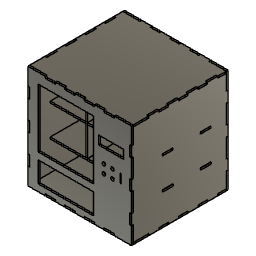
SAVEnding_CAD (Autodesk Fusion 360 design; units mm, degrees)
Autodesk Fusion 360 part; units mm, degrees
note: some values were not read from the file. Set by a fixed rule: which sketch regions a step uses.
(part 1 of 2)
sketch "Sketch3" plane through (0, 0, 0) normal (0, 1, 0) x (1, 0, 0)
  line L0 (0, 0) -> (300, 0)
  line L1 (300, 0) -> (300, -300)
  line L2 (300, -300) -> (0, -300)
  line L3 (0, -300) -> (0, 0)
  dimension "d9" = 300
  dimension "d10" = 300
  constraint horizontal L0
  constraint vertical L1
  constraint horizontal L2
  constraint vertical L3
  constraint coincident L0.start L3.end
  measures "d9" distance of L0.start L0.end
  measures "d10" distance of L0.start L2.end
extrude "Extrude2" add sketch "Sketch3" along normal blind 5 makes body 1
sketch "Sketch4" plane through (0, 0, 0) normal (0, 0, 1) x (1, 0, 0)
  line L0 (0, 0) -> (300, 0)
  line L1 (300, 0) -> (300, 280)
  line L2 (300, 280) -> (0, 280)
  line L3 (0, 280) -> (0, 0)
  dimension "d13" = 300
  dimension "d14" = 280
  constraint horizontal L0
  constraint vertical L1
  constraint horizontal L2
  constraint vertical L3
  constraint coincident L0.start L3.end
  measures "d13" distance of L0.start L0.end
  measures "d14" distance of L0.start L2.end
sketch "Sketch5" plane through (0, 0, 0) normal (0, 0, 1) x (1, 0, 0)
sketch "Sketch6" plane through (0, 0, 0) normal (0, 0, 1) x (1, 0, 0)
  line L0 (50, 0) -> (80, 0)
  line L1 (80, 0, 0) -> (80, 0, 5)
  line L2 (80, 0, 5) -> (50, 0, 5)
  line L3 (50, 0, 5) -> (50, 0, 0)
  line L4 (0, 0) -> (300, 0)
  dimension "d28" = 30
  dimension "d29" = 5
  constraint horizontal L0
  constraint coincident L0.start L4
  measures "d28" distance of L0.start L0.end
sketch "Sketch7" plane through (0, 0, 0) normal (0, 1, 0) x (1, 0, 0)
  line L0 (50, 0) -> (80, 0)
  line L1 (80, 0) -> (80, -5)
  line L2 (80, -5) -> (50, -5)
  line L3 (50, -5) -> (50, 0)
  dimension "d32" = 30
  dimension "d33" = 5
  constraint horizontal L0
  constraint vertical L1
  constraint horizontal L2
  constraint vertical L3
  measures "d32" distance of L0.start L0.end
  measures "d33" distance of L0.start L2.end
extrude "Extrude5" cut sketch "Sketch7" along normal blind 5 bodies 1
pattern_linear "R-Pattern1" count 1 spacing 0 along (0, 0, -1) count 4 spacing 56.6667 along (1, 0, 0) of "Extrude5"
ref_plane "WorkPlane1" through (150, 2.5, 150) normal (0, 0, 1) x (1, 0, 0)
mirror "Mirror1" about plane through (150, 2.5, 150) normal (0, 0, 1) of "Extrude5", "R-Pattern1"
sketch "Sketch8" plane through (0, 0, 0) normal (0, 0, 1) x (1, 0, 0)
  line L0 (0, 0) -> (300, 0)
  line L1 (300, 0) -> (300, 280)
  line L2 (300, 280) -> (0, 280)
  line L3 (0, 280) -> (0, 0)
  dimension "d42" = 300
  dimension "d43" = 280
  constraint horizontal L0
  constraint vertical L1
  constraint horizontal L2
  constraint vertical L3
  constraint coincident L0.start L3.end
  measures "d42" distance of L0.start L0.end
  measures "d43" distance of L0.start L2.end
extrude "Extrude6" add sketch "Sketch8" along normal blind 5 separate body makes body 2
combine "Combine1" operation cut target body 2 tool bodies 1 keep tools
sketch "Sketch9" plane through (0, 0, 0) normal (0, 0, 1) x (1, 0, 0)
  line L0 (0, 50) -> (5, 50)
  line L1 (5, 50) -> (5, 80)
  line L2 (5, 80) -> (0, 80)
  line L3 (0, 80) -> (0, 50)
  dimension "d48" = 5
  dimension "d49" = 30
  constraint horizontal L0
  constraint vertical L1
  constraint horizontal L2
  constraint vertical L3
  measures "d48" distance of L0.start L0.end
  measures "d49" distance of L0.start L2.end
extrude "Extrude7" cut sketch "Sketch9" along normal blind 5 bodies 2
pattern_linear "R-Pattern2" count 4 spacing 56.6667 along (0, 1, 0) of "Extrude7"
ref_plane "WorkPlane4" through (150, 140, 2.5) normal (-1, 0, 0) x (0, -1, 0)
mirror "Mirror3" about plane through (150, 140, 2.5) normal (-1, 0, 0) of "Extrude7", "R-Pattern2"
ref_plane "WorkPlane5" through (150, 2.5, 150) normal (0, 0, 1) x (1, 0, 0)
mirror "Mirror5" about plane through (150, 2.5, 150) normal (0, 0, 1) of bodies 2 makes body 3
sketch "Sketch10" plane through (0, 0, 0) normal (1, 0, 0) x (0, 1, 0)
  line L0 (0, 50) -> (5, 50)
  line L1 (5, 50) -> (5, 80)
  line L2 (5, 80) -> (0, 80)
  line L3 (0, 80) -> (0, 50)
  dimension "d63" = 5
  dimension "d64" = 30
  constraint horizontal L0
  constraint vertical L1
  constraint horizontal L2
  constraint vertical L3
  measures "d63" distance of L0.start L0.end
  measures "d64" distance of L0.start L2.end
extrude "Extrude8" cut sketch "Sketch10" along normal blind 5 bodies 1
pattern_linear "R-Pattern3" count 1 spacing 0 along (1, 0, 0) count 3 spacing 85 along (0, 0, 1) of "Extrude8"
ref_plane "WorkPlane6" through (150, 2.5, 150) normal (-1, 0, 0) x (0, 0, 1)
mirror "Mirror6" about plane through (150, 2.5, 150) normal (-1, 0, 0) of "Extrude8", "R-Pattern3"
ref_plane "WorkPlane7" through (150, 140, 150) normal (0, -1, 0) x (-1, 0, 0)
mirror "Mirror7" about plane through (150, 140, 150) normal (0, -1, 0) of bodies 1 makes body 4
combine "Combine2" operation cut target body 2 tool bodies 4 keep tools
combine "Combine3" operation cut target body 3 tool bodies 4 keep tools
sketch "Sketch11" plane through (0, 0, 0) normal (1, 0, 0) x (0, 1, 0)
  line L0 (0, 0) -> (280, 0)
  line L1 (280, 0) -> (280, 300)
  line L2 (280, 300) -> (0, 300)
  line L3 (0, 300) -> (0, 0)
  dimension "d75" = 280
  dimension "d76" = 300
  constraint horizontal L0
  constraint vertical L1
  constraint horizontal L2
  constraint vertical L3
  constraint coincident L0.start L3.end
  measures "d75" distance of L0.start L0.end
  measures "d76" distance of L0.start L2.end
extrude "Extrude9" add sketch "Sketch11" along normal blind 5 separate body makes body 5
combine "Combine4" operation cut target body 5 tool bodies 1 2 3 4 keep tools
mirror "Mirror8" about plane through (150, 2.5, 150) normal (-1, 0, 0) of bodies 5 makes body 6
sketch "Sketch12" plane through (0, 0, 0) normal (0, -1, 0) x (1, 0, 0)
  line L0 (295, 250) -> (300, 250)
  line L1 (300, 250) -> (300, 300)
  line L2 (250, 295) -> (220, 295)
  line L3 (220, 295) -> (220, 300)
  line L4 (300, 300) -> (250, 300)
  line L5 (193.3333, 300) -> (193.3333, 295)
  line L6 (193.3333, 295) -> (163.3333, 295)
  line L7 (163.3333, 295) -> (163.3333, 300)
  line L8 (163.3333, 300) -> (136.6667, 300)
  line L9 (136.6667, 300) -> (136.6667, 295)
  line L10 (136.6667, 295) -> (106.6667, 295)
  line L11 (106.6667, 295) -> (106.6667, 300)
  line L12 (106.6667, 300) -> (80, 300)
  line L13 (80, 300) -> (80, 295)
  line L14 (80, 295) -> (50, 295)
  line L15 (50, 295) -> (50, 300)
  line L16 (50, 300) -> (0, 300)
  line L17 (0, 300) -> (0, 250)
  line L18 (0, 250) -> (5, 250)
  line L19 (5, 250) -> (5, 220)
  line L20 (5, 220) -> (0, 220)
  line L21 (0, 220) -> (0, 165)
  line L22 (0, 165) -> (5, 165)
  line L23 (5, 165) -> (5, 135)
  line L24 (5, 135) -> (0, 135)
  line L25 (0, 135) -> (0, 80)
  line L26 (0, 80) -> (5, 80)
  line L27 (5, 80) -> (5, 50)
  line L28 (5, 50) -> (0, 50)
  line L29 (0, 50) -> (0, 0)
  line L30 (0, 0) -> (50, 0)
  line L31 (50, 0) -> (50, 5)
  line L32 (50, 5) -> (80, 5)
  line L33 (80, 5) -> (80, 0)
  line L34 (80, 0) -> (106.6667, 0)
  line L35 (106.6667, 0) -> (106.6667, 5)
  line L36 (106.6667, 5) -> (136.6667, 5)
  line L37 (136.6667, 5) -> (136.6667, 0)
  line L38 (136.6667, 0) -> (163.3333, 0)
  line L39 (163.3333, 0) -> (163.3333, 5)
  line L40 (163.3333, 5) -> (193.3333, 5)
  line L41 (193.3333, 5) -> (193.3333, 0)
  line L42 (193.3333, 0) -> (220, 0)
  line L43 (220, 0) -> (220, 5)
  line L44 (220, 5) -> (250, 5)
  line L45 (300, 50) -> (295, 50)
  line L46 (295, 50) -> (295, 80)
  line L47 (295, 80) -> (300, 80)
  line L48 (300, 80) -> (300, 135)
  line L49 (300, 135) -> (295, 135)
  line L50 (295, 135) -> (295, 165)
  line L51 (295, 165) -> (300, 165)
  line L52 (300, 165) -> (300, 220)
  line L53 (300, 220) -> (295, 220)
  line L54 (295, 220) -> (295, 250)
  line L55 (30, 20) -> (190, 20)
  line L56 (190, 20) -> (190, 80)
  line L57 (190, 80) -> (30, 80)
  line L58 (30, 80) -> (30, 20)
  line L59 (250, 300) -> (250, 295)
  line L60 (250, 5) -> (250, 0)
  line L61 (250, 0) -> (300, 0)
  line L62 (300, 0) -> (300, 50)
  line L63 (220, 300) -> (193.3333, 300)
  dimension "d81" = 160
  dimension "d82" = 60
  constraint horizontal L55
  constraint vertical L56
  constraint horizontal L57
  constraint vertical L58
  measures "d81" distance of L55.start L55.end
  measures "d82" distance of L55.start L57.end
extrude "Extrude10" cut sketch "Sketch12" against normal blind 5 contours L55 L56 L57 L58 bodies 1
sketch "Sketch13" plane through (0, 0, 0) normal (0, -1, 0) x (1, 0, 0)
  line L0 (190, 20) -> (30, 20)
  line L1 (30, 20) -> (30, 80)
  line L2 (30, 80) -> (190, 80)
  line L3 (190, 80) -> (190, 20)
  line L4 (295, 250) -> (300, 250)
  line L5 (300, 250) -> (300, 300)
  line L6 (250, 295) -> (220, 295)
  line L7 (220, 295) -> (220, 300)
  line L8 (300, 300) -> (250, 300)
  line L9 (193.3333, 300) -> (193.3333, 295)
  line L10 (193.3333, 295) -> (163.3333, 295)
  line L11 (163.3333, 295) -> (163.3333, 300)
  line L12 (163.3333, 300) -> (136.6667, 300)
  line L13 (136.6667, 300) -> (136.6667, 295)
  line L14 (136.6667, 295) -> (106.6667, 295)
  line L15 (106.6667, 295) -> (106.6667, 300)
  line L16 (106.6667, 300) -> (80, 300)
  line L17 (80, 300) -> (80, 295)
  line L18 (80, 295) -> (50, 295)
  line L19 (50, 295) -> (50, 300)
  line L20 (50, 300) -> (0, 300)
  line L21 (0, 300) -> (0, 250)
  line L22 (0, 250) -> (5, 250)
  line L23 (5, 250) -> (5, 220)
  line L24 (5, 220) -> (0, 220)
  line L25 (0, 220) -> (0, 165)
  line L26 (0, 165) -> (5, 165)
  line L27 (5, 165) -> (5, 135)
  line L28 (5, 135) -> (0, 135)
  line L29 (0, 135) -> (0, 80)
  line L30 (0, 80) -> (5, 80)
  line L31 (5, 80) -> (5, 50)
  line L32 (5, 50) -> (0, 50)
  line L33 (0, 50) -> (0, 0)
  line L34 (0, 0) -> (50, 0)
  line L35 (50, 0) -> (50, 5)
  line L36 (50, 5) -> (80, 5)
  line L37 (80, 5) -> (80, 0)
  line L38 (80, 0) -> (106.6667, 0)
  line L39 (106.6667, 0) -> (106.6667, 5)
  line L40 (106.6667, 5) -> (136.6667, 5)
  line L41 (136.6667, 5) -> (136.6667, 0)
  line L42 (136.6667, 0) -> (163.3333, 0)
  line L43 (163.3333, 0) -> (163.3333, 5)
  line L44 (163.3333, 5) -> (193.3333, 5)
  line L45 (193.3333, 5) -> (193.3333, 0)
  line L46 (193.3333, 0) -> (220, 0)
  line L47 (220, 0) -> (220, 5)
  line L48 (220, 5) -> (250, 5)
  line L49 (300, 50) -> (295, 50)
  line L50 (295, 50) -> (295, 80)
  line L51 (295, 80) -> (300, 80)
  line L52 (300, 80) -> (300, 135)
  line L53 (300, 135) -> (295, 135)
  line L54 (295, 135) -> (295, 165)
  line L55 (295, 165) -> (300, 165)
  line L56 (300, 165) -> (300, 220)
  line L57 (300, 220) -> (295, 220)
  line L58 (295, 220) -> (295, 250)
  line L59 (30, 100) -> (190, 100)
  line L60 (190, 100) -> (190, 270)
  line L61 (190, 270) -> (30, 270)
  line L62 (30, 270) -> (30, 100)
  line L63 (250, 300) -> (250, 295)
  line L64 (250, 5) -> (250, 0)
  line L65 (250, 0) -> (300, 0)
  line L66 (300, 0) -> (300, 50)
  line L67 (220, 300) -> (193.3333, 300)
  dimension "d85" = 160
  dimension "d86" = 170
  constraint horizontal L59
  constraint vertical L60
  constraint horizontal L61
  constraint vertical L62
  measures "d85" distance of L59.start L59.end
  measures "d86" distance of L59.start L61.end
extrude "Extrude11" cut sketch "Sketch13" against normal blind 5 contours L59 L60 L61 L62 bodies 1
sketch "Sketch18" plane through (0, 0, 0) normal (0, 0, 1) x (1, 0, 0)
  line L0 (310, 260) -> (600, 260)
  line L1 (600, 260) -> (600, 60)
  line L2 (600, 60) -> (310, 60)
  line L3 (310, 60) -> (310, 260)
  line L4 (310, 230) -> (304, 230)
  line L5 (304, 230) -> (304, 200)
  line L6 (304, 200) -> (310, 200)
  line L7 (310, 200) -> (310, 230)
  line L8 (310, 90) -> (304, 90)
  line L9 (304, 90) -> (304, 120)
  line L10 (304, 120) -> (310, 120)
  line L11 (310, 120) -> (310, 90)
  line L12 (600, 230) -> (606, 230)
  line L13 (606, 230) -> (606, 200)
  line L14 (606, 200) -> (600, 200)
  line L15 (600, 200) -> (600, 230)
  line L16 (600, 90) -> (606, 90)
  line L17 (606, 90) -> (606, 120)
  line L18 (606, 120) -> (600, 120)
  line L19 (600, 120) -> (600, 90)
  dimension "d115" = 290
  dimension "d116" = 200
  dimension "d117" = 6
  dimension "d118" = 30
  dimension "d119" = 6
  dimension "d120" = 30
  dimension "d121" = 6
  dimension "d122" = 30
  dimension "d123" = 6
  dimension "d124" = 30
  constraint horizontal L0
  constraint vertical L1
  constraint horizontal L2
  constraint vertical L3
  constraint horizontal L4
  constraint vertical L5
  constraint horizontal L6
  constraint vertical L7
  constraint coincident L3 L4.start
  constraint horizontal L8
  constraint vertical L9
  constraint horizontal L10
  constraint vertical L11
  constraint coincident L3 L8.start
  constraint horizontal L12
  constraint vertical L13
  constraint horizontal L14
  constraint vertical L15
  constraint coincident L1 L12.start
  constraint horizontal L16
  constraint vertical L17
  constraint horizontal L18
  constraint vertical L19
  constraint coincident L1 L16.start
  measures "d115" distance of L0.start L0.end
  measures "d116" distance of L0.start L2.end
  measures "d117" distance of L4.start L4.end
  measures "d118" distance of L4.start L6.end
  measures "d119" distance of L8.start L8.end
  measures "d120" distance of L8.start L10.end
  measures "d121" distance of L12.start L12.end
  measures "d122" distance of L12.start L14.end
  measures "d123" distance of L16.start L16.end
  measures "d124" distance of L16.start L18.end
extrude "Extrude15" add sketch "Sketch18" along normal blind 5 separate body makes body 7
copy_body "CopyPasteBodies1" bodies 7 makes body 8
move_body "Move2" bodies 8 to x (1, 0, 0) y (0, 1, 0) z (0, 0, 1) at (0, 0, 90)
move_body "Move3" bodies 7 8 to x (1, 0, 0) y (0, 1, 0) z (0, 0, 1) at (-305, 0, 90)
combine "Combine8" operation cut target body 6 tool bodies 8 7 keep tools
combine "Combine9" operation cut target body 5 tool bodies 8 7 keep tools
move_body "Move4" bodies 7 8 to x (1, 0, 0) y (0, 1, 0) z (0, 0, 1) at (320, 0, 0)
sketch "Sketch19" plane through (0, 0, 95) normal (0, 0, 1) x (-1, 0, 0)
  line L0 (-615, -90) -> (-621, -90)
  line L1 (-621, -90) -> (-621, -120)
  line L2 (-621, -120) -> (-615, -120)
  line L3 (-615, -120) -> (-615, -200)
  line L4 (-615, -200) -> (-621, -200)
  line L5 (-621, -200) -> (-621, -230)
  line L6 (-621, -230) -> (-615, -230)
  line L7 (-615, -230) -> (-615, -260)
  line L8 (-615, -260) -> (-325, -260)
  line L9 (-325, -260) -> (-325, -230)
  line L10 (-325, -230) -> (-319, -230)
  line L11 (-319, -230) -> (-319, -200)
  line L12 (-319, -200) -> (-325, -200)
  line L13 (-325, -200) -> (-325, -120)
  line L14 (-325, -120) -> (-319, -120)
  line L15 (-319, -120) -> (-319, -90)
  line L16 (-319, -90) -> (-325, -90)
  line L17 (-325, -90) -> (-325, -60)
  line L18 (-325, -60) -> (-615, -60)
  line L19 (-615, -60) -> (-615, -90)
  line L20 (-472.0378, -260) -> (-467.0378, -260)
  line L21 (-467.0378, -260) -> (-467.0378, -60)
  line L22 (-467.0378, -60) -> (-472.0378, -60)
  line L23 (-472.0378, -60) -> (-472.0378, -260)
  dimension "d127" = 5
  dimension "d128" = 200
  constraint horizontal L20
  constraint vertical L21
  constraint horizontal L22
  constraint vertical L23
  constraint coincident L8 L20.start
  measures "d127" distance of L20.start L20.end
  measures "d128" distance of L20.start L22.end
extrude "Extrude16" add sketch "Sketch19" along normal up to surface (85 mm away) separate body contours L8 L18 L20 L21 L22 L23 makes body 9
sketch "Sketch20" plane through (472.0378, 0, 0) normal (1, 0, 0) x (0, 1, 0)
  line L0 (260, 180) -> (60, 180)
  line L1 (60, 180) -> (60, 95)
  line L2 (60, 95) -> (260, 95)
  line L3 (260, 95) -> (260, 180)
  line L4 (90, 180) -> (120, 180)
  line L5 (120, 180) -> (120, 185)
  line L6 (120, 185) -> (90, 185)
  line L7 (90, 185) -> (90, 180)
  line L8 (200, 180) -> (230, 180)
  line L9 (230, 180) -> (230, 185)
  line L10 (230, 185) -> (200, 185)
  line L11 (200, 185) -> (200, 180)
  line L12 (90.0251, 95) -> (120.0251, 95)
  line L13 (120.0251, 95) -> (120.0251, 90)
  line L14 (120.0251, 90) -> (90.0251, 90)
  line L15 (90.0251, 90) -> (90.0251, 95)
  line L16 (200, 95) -> (230, 95)
  line L17 (230, 95) -> (230, 90)
  line L18 (230, 90) -> (200, 90)
  line L19 (200, 90) -> (200, 95)
  line L20 (260, 95) -> (60, 95)
  line L21 (60, 95) -> (60, 180)
  line L22 (60, 180) -> (260, 180)
  line L23 (260, 180) -> (260, 95)
  line L24 (60, 180) -> (260, 180)
  line L25 (260, 180) -> (260, 95)
  line L26 (260, 95) -> (60, 95)
  line L27 (60, 95) -> (60, 180)
  line L28 (60, 185) -> (260, 185)
  line L29 (260, 185) -> (260, 265)
  line L30 (260, 265) -> (60, 265)
  line L31 (60, 265) -> (60, 185)
  dimension "d131" = 30
  dimension "d132" = 5
  dimension "d133" = 30
  dimension "d134" = 5
  dimension "d135" = 30
  dimension "d136" = 5
  dimension "d137" = 30
  dimension "d138" = 5
  dimension "d139" = 200
  dimension "d140" = 80
  constraint horizontal L4
  constraint vertical L5
  constraint horizontal L6
  constraint vertical L7
  constraint coincident L0 L4.start
  constraint horizontal L8
  constraint vertical L9
  constraint horizontal L10
  constraint vertical L11
  constraint coincident L0 L8.start
  constraint horizontal L12
  constraint vertical L13
  constraint horizontal L14
  constraint vertical L15
  constraint coincident L2 L12.start
  constraint horizontal L16
  constraint vertical L17
  constraint horizontal L18
  constraint vertical L19
  constraint coincident L2 L16.start
  constraint horizontal L20
  constraint vertical L21
  constraint horizontal L22
  constraint vertical L23
  constraint coincident L0.end L1.start
  constraint coincident L2.end L3.start
  constraint horizontal L24
  constraint vertical L25
  constraint horizontal L26
  constraint vertical L27
  constraint horizontal L28
  constraint vertical L29
  constraint horizontal L30
  constraint vertical L31
  measures "d131" distance of L4.start L4.end
  measures "d132" distance of L4.start L6.end
  measures "d133" distance of L8.start L8.end
  measures "d134" distance of L8.start L10.end
  measures "d135" distance of L12.start L12.end
  measures "d136" distance of L12.start L14.end
  measures "d137" distance of L16.start L16.end
  measures "d138" distance of L16.start L18.end
  measures "d139" distance of L28.start L28.end
  measures "d140" distance of L28.start L30.end
extrude "Extrude17" add sketch "Sketch20" against normal blind 5 contours L0 L8 L9 L10 L11 L22 L24 L28 | L6 L10 L28 L29 L30 L31 | L2 L16 L17 L18 L19 L20 L26 | L0 L4 L5 L6 L7 L22 L24 L28 | L2 L12 L13 L14 L15 L20 L26 bodies 9
ref_plane "WorkPlane8" through (470, 160, 182.5) normal (0, -1, 0) x (1, 0, 0)
split "Split1" by plane through (470, 160, 182.5) normal (0, -1, 0) bodies 8 7 makes body 11 at (421.6667, 146.6667, 90) makes body 10 at (421.6667, 146.6667, 180)
move_body "Move5" bodies 9 to x (1, 0, 0) y (0, 1, 0) z (0, 0, 1) at (-40, 0, 0)
combine "Combine10" operation cut target body 8 tool bodies 9 keep tools
combine "Combine11" operation cut target body 10 tool bodies 9 keep tools
combine "Combine12" operation cut target body 7 tool bodies 9 keep tools
combine "Combine13" operation cut target body 11 tool bodies 9 keep tools
move_body "Move6" bodies 8 10 9 7 11 to x (1, 0, 0) y (0, 1, 0) z (0, 0, 1) at (-320, 0, 0)
sketch "Sketch21" plane through (0, 0, 0) normal (0, -1, 0) x (1, 0, 0)
  line L0 (190, 100) -> (30, 100)
  line L1 (30, 100) -> (30, 270)
  line L2 (30, 270) -> (190, 270)
  line L3 (190, 270) -> (190, 100)
  line L4 (190, 20) -> (30, 20)
  line L5 (30, 20) -> (30, 80)
  line L6 (30, 80) -> (190, 80)
  line L7 (190, 80) -> (190, 20)
  line L8 (295, 250) -> (300, 250)
  line L9 (300, 250) -> (300, 300)
  line L10 (250, 295) -> (220, 295)
  line L11 (220, 295) -> (220, 300)
  line L12 (300, 300) -> (250, 300)
  line L13 (193.3333, 300) -> (193.3333, 295)
  line L14 (193.3333, 295) -> (163.3333, 295)
  line L15 (163.3333, 295) -> (163.3333, 300)
  line L16 (163.3333, 300) -> (136.6667, 300)
  line L17 (136.6667, 300) -> (136.6667, 295)
  line L18 (136.6667, 295) -> (106.6667, 295)
  line L19 (106.6667, 295) -> (106.6667, 300)
  line L20 (106.6667, 300) -> (80, 300)
  line L21 (80, 300) -> (80, 295)
  line L22 (80, 295) -> (50, 295)
  line L23 (50, 295) -> (50, 300)
  line L24 (50, 300) -> (0, 300)
  line L25 (0, 300) -> (0, 250)
  line L26 (0, 250) -> (5, 250)
  line L27 (5, 250) -> (5, 220)
  line L28 (5, 220) -> (0, 220)
  line L29 (0, 220) -> (0, 165)
  line L30 (0, 165) -> (5, 165)
  line L31 (5, 165) -> (5, 135)
  line L32 (5, 135) -> (0, 135)
  line L33 (0, 135) -> (0, 80)
  line L34 (0, 80) -> (5, 80)
  line L35 (5, 80) -> (5, 50)
  line L36 (5, 50) -> (0, 50)
  line L37 (0, 50) -> (0, 0)
  line L38 (0, 0) -> (50, 0)
  line L39 (50, 0) -> (50, 5)
  line L40 (50, 5) -> (80, 5)
  line L41 (80, 5) -> (80, 0)
  line L42 (80, 0) -> (106.6667, 0)
  line L43 (106.6667, 0) -> (106.6667, 5)
  line L44 (106.6667, 5) -> (136.6667, 5)
  line L45 (136.6667, 5) -> (136.6667, 0)
  line L46 (136.6667, 0) -> (163.3333, 0)
  line L47 (163.3333, 0) -> (163.3333, 5)
  line L48 (163.3333, 5) -> (193.3333, 5)
  line L49 (193.3333, 5) -> (193.3333, 0)
  line L50 (193.3333, 0) -> (220, 0)
  line L51 (220, 0) -> (220, 5)
  line L52 (220, 5) -> (250, 5)
  line L53 (300, 50) -> (295, 50)
  line L54 (295, 50) -> (295, 80)
  line L55 (295, 80) -> (300, 80)
  line L56 (300, 80) -> (300, 135)
  line L57 (300, 135) -> (295, 135)
  line L58 (295, 135) -> (295, 165)
  line L59 (295, 165) -> (300, 165)
  line L60 (300, 165) -> (300, 220)
  line L61 (300, 220) -> (295, 220)
  line L62 (295, 220) -> (295, 250)
  line L63 (205, 230) -> (277, 230)
  line L64 (277, 230) -> (277, 205)
  line L65 (277, 205) -> (205, 205)
  line L66 (205, 205) -> (205, 230)
  line L67 (267.4, 165) -> (270, 165)
  line L68 (270, 165) -> (270, 140)
  line L69 (270, 140) -> (267.4, 140)
  line L70 (267.4, 140) -> (267.4, 165)
  circle A0 centre (220, 140) radius 5
  circle A1 centre (245, 140) radius 5
  circle A2 centre (220, 165) radius 5
  circle A3 centre (245, 165) radius 5
  line L71 (250, 300) -> (250, 295)
  line L72 (250, 5) -> (250, 0)
  line L73 (250, 0) -> (300, 0)
  line L74 (300, 0) -> (300, 50)
  line L75 (220, 300) -> (193.3333, 300)
  dimension "d143" = 72
  dimension "d144" = 25
  dimension "d145" = 2.6
  dimension "d146" = 25
  dimension "d147" = 10
  dimension "d148" = 10
  dimension "d149" = 10
  dimension "d150" = 10
  constraint horizontal L63
  constraint vertical L64
  constraint horizontal L65
  constraint vertical L66
  constraint horizontal L67
  constraint vertical L68
  constraint horizontal L69
  constraint vertical L70
  measures "d143" distance of L63.start L63.end
  measures "d144" distance of L63.start L65.end
  measures "d145" distance of L67.start L67.end
  measures "d146" distance of L67.start L69.end
  measures "d147" diameter of A0
  measures "d148" diameter of A1
  measures "d149" diameter of A2
  measures "d150" diameter of A3
extrude "Extrude18" cut sketch "Sketch21" against normal blind 5 contours L63 L64 L65 L66 | L67 L68 L69 L70 | A0 | A1 | A2 | A3 bodies 1
move_body "Move7" bodies 9 to x (1, 0, 0) y (0, 1, 0) z (0, 0, 1) at (0, 250, 0)
sketch "Sketch22" plane through (0, 510, 0) normal (0, 1, 0) x (-1, 0, 0)
  line L0 (-112.0378, 265) -> (-112.0378, 185)
  line L1 (-112.0378, 185) -> (-107.0378, 185)
  line L2 (-107.0378, 185) -> (-107.0378, 265)
  line L3 (-107.0378, 265) -> (-112.0378, 265)
  line L4 (-50, 240) -> (-170, 240)
  line L5 (-170, 240) -> (-170, 110)
  line L6 (-170, 110) -> (-50, 110)
  line L7 (-50, 110) -> (-50, 240)
  dimension "d153" = 120
  dimension "d154" = 130
  constraint horizontal L4
  constraint vertical L5
  constraint horizontal L6
  constraint vertical L7
  measures "d153" distance of L4.start L4.end
  measures "d154" distance of L4.start L6.end
extrude "Extrude19" add sketch "Sketch22" along normal blind 5 separate body contours L0 L1 L2 L4 | L0 L1 L2 L4 L5 L6 L7 makes body 12
sketch "Sketch23" plane through (0, 515, 0) normal (0, 1, 0) x (-1, 0, 0)
  line L0 (-50, 110) -> (-50, 240)
  line L1 (-50, 240) -> (-170, 240)
  line L2 (-170, 240) -> (-170, 110)
  line L3 (-170, 110) -> (-50, 110)
  line L4 (-63.5, 222.5) -> (-76.5, 222.5)
  line L5 (-76.5, 222.5) -> (-76.5, 197.5)
  line L6 (-76.5, 197.5) -> (-63.5, 197.5)
  line L7 (-63.5, 197.5) -> (-63.5, 222.5)
  line L8 (-63.5, 222.5) -> (-76.5, 197.5) construction
  line L9 (-76.5, 222.5) -> (-63.5, 197.5) construction
  line L10 (-156.5, 222.5) -> (-156.5, 197.5)
  line L11 (-143.5, 222.5) -> (-156.5, 222.5)
  line L12 (-143.5, 197.5) -> (-143.5, 222.5)
  line L13 (-156.5, 197.5) -> (-143.5, 197.5)
  line L14 (-76.5, 142.5) -> (-76.5, 117.5)
  line L15 (-63.5, 142.5) -> (-76.5, 142.5)
  line L16 (-63.5, 117.5) -> (-63.5, 142.5)
  line L17 (-76.5, 117.5) -> (-63.5, 117.5)
  line L18 (-156.5, 142.5) -> (-156.5, 117.5)
  line L19 (-143.5, 142.5) -> (-156.5, 142.5)
  line L20 (-143.5, 117.5) -> (-143.5, 142.5)
  line L21 (-156.5, 117.5) -> (-143.5, 117.5)
  point P0 (-70, 210)
  dimension "d157" = 13
  dimension "d158" = 25
  dimension "d161" = -80
  dimension "d162" = -80
  constraint horizontal L4
  constraint perpendicular L4 L5
  constraint parallel L4 L6
  constraint parallel L5 L7
  constraint coincident L8 P0
  constraint coincident L9 P0
  measures "d157" distance of L5.end L6.end
  measures "d158" distance of L4.end L5.end
extrude "Extrude20" cut sketch "Sketch23" against normal blind 5 contours L4 L5 L6 L7 | L10 L11 L12 L13 | L14 L15 L16 L17 | L18 L19 L20 L21 bodies 12
sketch "Sketch24" plane through (112.0378, 0, 0) normal (1, 0, 0) x (0, 1, 0)
  line L0 (340, 180) -> (310, 180)
  line L1 (310, 180) -> (310, 95)
  line L2 (310, 95) -> (340.0251, 95)
  line L3 (340.0251, 95) -> (340.0251, 90)
  line L4 (340.0251, 90) -> (370.0251, 90)
  line L5 (370.0251, 90) -> (370.0251, 95)
  line L6 (370.0251, 95) -> (450, 95)
  line L7 (450, 95) -> (450, 90)
  line L8 (450, 90) -> (480, 90)
  line L9 (480, 90) -> (480, 95)
  line L10 (480, 95) -> (510, 95)
  line L11 (510, 95) -> (510, 180)
  line L12 (510, 180) -> (480, 180)
  line L13 (480, 180) -> (480, 185)
  line L14 (340, 185) -> (340, 180)
  line L15 (370, 180) -> (370, 185)
  line L16 (450, 185) -> (450, 180)
  line L17 (450, 180) -> (370, 180)
  line L18 (510, 225) -> (516, 225)
  line L19 (516, 225) -> (516, 195)
  line L20 (516, 195) -> (510, 195)
  line L21 (510, 195) -> (510, 225)
  line L22 (510, 125) -> (516, 125)
  line L23 (516, 125) -> (516, 155)
  line L24 (516, 155) -> (510, 155)
  line L25 (510, 155) -> (510, 125)
  line L26 (480, 185) -> (510, 185)
  line L27 (510, 185) -> (510, 265)
  line L28 (510, 265) -> (310, 265)
  line L29 (310, 265) -> (310, 185)
  line L30 (310, 185) -> (340, 185)
  line L31 (370, 185) -> (450, 185)
  dimension "d165" = 6
  dimension "d166" = 30
  dimension "d167" = 6
  dimension "d168" = 30
  constraint horizontal L18
  constraint vertical L19
  constraint horizontal L20
  constraint vertical L21
  constraint horizontal L22
  constraint vertical L23
  constraint horizontal L24
  constraint vertical L25
  constraint coincident L11 L22.start
  measures "d165" distance of L18.start L18.end
  measures "d166" distance of L18.start L20.end
  measures "d167" distance of L22.start L22.end
  measures "d168" distance of L22.start L24.end
extrude "Extrude21" add sketch "Sketch24" against normal blind 5 contours L18 L19 L20 L21 L27 | L11 L22 L23 L24 L25 bodies 9
combine "Combine14" operation cut target body 12 tool bodies 9 keep tools
move_body "Move8" bodies 12 9 to x (1, 0, 0) y (0, 1, 0) z (0, 0, 1) at (0, -250, 0)
ref_plane "WorkPlane9" through (412.0378, 163, 177.5) normal (1, 0, 0) x (0, 1, 0)
sketch "Sketch25" plane through (412.0378, 163, 177) normal (1, 0, 0) x (0, 1, 0)
  line L0 (-125, 75) -> (55, 75)
  line L1 (55, 75) -> (55, -5)
  line L2 (55, -5) -> (-125, -5)
  line L3 (-125, -5) -> (-125, 75)
  line L4 (-125, -10) -> (55, -10)
  line L5 (55, -10) -> (55, -96)
  line L6 (-125, -96) -> (-125, -10)
  line L7 (4.9998, -5) -> (-55.0002, -5)
  line L8 (-55.0002, -5) -> (-55.0002, -10)
  line L9 (-55.0002, -10) -> (4.9998, -10)
  line L10 (4.9998, -10) -> (4.9998, -5)
  line L11 (4.9998, -5) -> (-55.0002, -10) construction
  line L12 (-55.0002, -5) -> (4.9998, -10) construction
  line L13 (55, 6) -> (60, 6)
  line L14 (60, 6) -> (60, 36)
  line L15 (60, 36) -> (55, 36)
  line L16 (55, 36) -> (55, 6)
  line L17 (55, -20) -> (60, -20)
  line L18 (60, -20) -> (60, -50)
  line L19 (60, -50) -> (55, -50)
  line L20 (55, -50) -> (55, -20)
  line L21 (-125, -96) -> (55, -96)
  line L22 (-65, -96) -> (-65, -101)
  line L23 (-65, -101) -> (-95, -101)
  line L24 (-95, -101) -> (-95, -96)
  line L25 (-95, -96) -> (-125, -96)
  line L26 (45, -96) -> (45, -101)
  line L27 (45, -101) -> (15, -101)
  line L28 (15, -101) -> (15, -96)
  line L29 (55, -96) -> (45, -96)
  line L30 (15, -96) -> (-65, -96)
  point P0 (-25.0002, -7.5)
  dimension "d172" = 180
  dimension "d173" = 80
  dimension "d174" = 180
  dimension "d175" = 86
  dimension "d176" = 60
  dimension "d177" = 5
  dimension "d178" = 5
  dimension "d179" = 30
  dimension "d180" = 5
  dimension "d181" = 30
  dimension "d182" = 180
  dimension "d194" = 30
  dimension "d195" = 5
  dimension "d198" = 110
  dimension "d199" = 0
  constraint horizontal L0
  constraint vertical L1
  constraint horizontal L2
  constraint vertical L3
  constraint horizontal L4
  constraint vertical L5
  constraint horizontal L29
  constraint vertical L6
  constraint horizontal L7
  constraint perpendicular L7 L8
  constraint parallel L7 L9
  constraint parallel L8 L10
  constraint coincident L11 P0
  constraint coincident L12 P0
  constraint coincident L2 L7.start
  constraint horizontal L13
  constraint vertical L14
  constraint horizontal L15
  constraint vertical L16
  constraint coincident L1 L13.start
  constraint horizontal L17
  constraint vertical L18
  constraint horizontal L19
  constraint vertical L20
  constraint coincident L5 L17.start
  constraint horizontal L21
  constraint vertical L22
  constraint horizontal L23
  constraint vertical L24
  constraint coincident L24.end L29
  constraint collinear L25 L29
  constraint collinear L29 L30
  measures "d172" distance of L0.start L0.end
  measures "d173" distance of L0.start L2.end
  measures "d174" distance of L4.start L4.end
  measures "d175" distance of L4.start L6.start
  measures "d176" distance of L8.end L9.end
  measures "d177" distance of L7.end L8.end
  measures "d178" distance of L13.start L13.end
  measures "d179" distance of L13.start L15.end
  measures "d180" distance of L17.start L17.end
  measures "d181" distance of L17.start L19.end
  measures "d182" distance of L6.start L5.end
  measures "d194" distance of L24.end L22.start
  measures "d195" distance of L24.end L23.end
extrude "Extrude22" add sketch "Sketch25" along normal blind 5 separate body contours L0 L1 L2 L3 L7 L16 | L1 L13 L14 L15 L16 | L2 L4 L7 L8 L9 L10 | L4 L5 L6 L9 L20 L21 L25 L29 L30 | L5 L17 L18 L19 L20 makes body 13
move_body "Move9" bodies 13 to x (1, 0, 0) y (0, 1, 0) z (0, 0, 1) at (-304, 22, 13)
combine "Combine15" operation cut target body 13 tool bodies 11 7 keep tools
sketch "Sketch26" plane through (0, 0, 0) normal (0, 0, 1) x (1, 0, 0)
  line L0 (310, 240) -> (610, 240)
  line L1 (610, 240) -> (610, 160)
  line L2 (610, 160) -> (310, 160)
  line L3 (310, 160) -> (310, 240)
  dimension "d186" = 300
  dimension "d187" = 80
  constraint horizontal L0
  constraint vertical L1
  constraint horizontal L2
  constraint vertical L3
  measures "d186" distance of L0.start L0.end
  measures "d187" distance of L0.start L2.end
extrude "Extrude23" add sketch "Sketch26" along normal blind 5 separate body makes body 14
move_body "Move10" bodies 14 to x (1, 0, 0) y (0, 1, 0) z (0, 0, 1) at (-310, 0, 180)
combine "Combine16" operation cut target body 14 tool bodies 13 6 5 keep tools
sketch "Sketch27" plane through (0, 0, 0) normal (0, 0, 1) x (1, 0, 0)
  line L0 (310, 60) -> (610, 60)
  line L1 (610, 60) -> (610, 160)
  line L2 (610, 160) -> (310, 160)
  line L3 (310, 160) -> (310, 60)
  dimension "d190" = 300
  dimension "d191" = 100
  constraint horizontal L0
  constraint vertical L1
  constraint horizontal L2
  constraint vertical L3
  measures "d190" distance of L0.start L0.end
  measures "d191" distance of L0.start L2.end
extrude "Extrude24" add sketch "Sketch27" along normal blind 5 separate body makes body 15
move_body "Move11" bodies 15 to x (1, 0, 0) y (0, 1, 0) z (0, 0, 1) at (-310, 0, 180)
combine "Combine17" operation cut target body 15 tool bodies 5 13 6 keep tools
move_body "Move12" bodies 12 to x (1, 0, 0) y (0, 1, 0) z (0, 0, 1) at (0, -20, 0)
sketch "front" plane through (0, 0, 0) normal (0, -1, 0) x (1, 0, 0)
  circle A0 centre (245, 140) radius 5
  line L0 (277, 230) -> (277, 205)
  line L1 (277, 205) -> (205, 205)
  line L2 (205, 205) -> (205, 230)
  line L3 (205, 230) -> (277, 230)
  circle A1 centre (220, 140) radius 5
  circle A2 centre (245, 165) radius 5
  circle A3 centre (220, 165) radius 5
  line L4 (270, 165) -> (270, 140)
  line L5 (270, 140) -> (267.4, 140)
  line L6 (267.4, 140) -> (267.4, 165)
  line L7 (267.4, 165) -> (270, 165)
  line L8 (190, 100) -> (30, 100)
  line L9 (30, 100) -> (30, 270)
  line L10 (30, 270) -> (190, 270)
  line L11 (190, 270) -> (190, 100)
  line L12 (190, 20) -> (30, 20)
  line L13 (30, 20) -> (30, 80)
  line L14 (30, 80) -> (190, 80)
  line L15 (190, 80) -> (190, 20)
  line L16 (295, 250) -> (300, 250)
  line L17 (300, 250) -> (300, 300)
  line L18 (300, 300) -> (250, 300)
  line L19 (250, 300) -> (250, 295)
  line L20 (250, 295) -> (220, 295)
  line L21 (220, 295) -> (220, 300)
  line L22 (220, 300) -> (193.3333, 300)
  line L23 (193.3333, 300) -> (193.3333, 295)
  line L24 (193.3333, 295) -> (163.3333, 295)
  line L25 (163.3333, 295) -> (163.3333, 300)
  line L26 (163.3333, 300) -> (136.6667, 300)
  line L27 (136.6667, 300) -> (136.6667, 295)
  line L28 (136.6667, 295) -> (106.6667, 295)
  line L29 (106.6667, 295) -> (106.6667, 300)
  line L30 (106.6667, 300) -> (80, 300)
  line L31 (80, 300) -> (80, 295)
  line L32 (80, 295) -> (50, 295)
  line L33 (50, 295) -> (50, 300)
  line L34 (50, 300) -> (0, 300)
  line L35 (0, 300) -> (0, 250)
  line L36 (0, 250) -> (5, 250)
  line L37 (5, 250) -> (5, 220)
  line L38 (5, 220) -> (0, 220)
  line L39 (0, 220) -> (0, 165)
  line L40 (0, 165) -> (5, 165)
  line L41 (5, 165) -> (5, 135)
  line L42 (5, 135) -> (0, 135)
  line L43 (0, 135) -> (0, 80)
  line L44 (0, 80) -> (5, 80)
  line L45 (5, 80) -> (5, 50)
  line L46 (5, 50) -> (0, 50)
  line L47 (0, 50) -> (0, 0)
  line L48 (0, 0) -> (50, 0)
  line L49 (50, 0) -> (50, 5)
  line L50 (50, 5) -> (80, 5)
  line L51 (80, 5) -> (80, 0)
  line L52 (80, 0) -> (106.6667, 0)
  line L53 (106.6667, 0) -> (106.6667, 5)
  line L54 (106.6667, 5) -> (136.6667, 5)
  line L55 (136.6667, 5) -> (136.6667, 0)
  line L56 (136.6667, 0) -> (163.3333, 0)
  line L57 (163.3333, 0) -> (163.3333, 5)
  line L58 (163.3333, 5) -> (193.3333, 5)
  line L59 (193.3333, 5) -> (193.3333, 0)
  line L60 (193.3333, 0) -> (220, 0)
  line L61 (220, 0) -> (220, 5)
  line L62 (220, 5) -> (250, 5)
  line L63 (250, 5) -> (250, 0)
  line L64 (250, 0) -> (300, 0)
  line L65 (300, 0) -> (300, 50)
  line L66 (300, 50) -> (295, 50)
  line L67 (295, 50) -> (295, 80)
  line L68 (295, 80) -> (300, 80)
  line L69 (300, 80) -> (300, 135)
  line L70 (300, 135) -> (295, 135)
  line L71 (295, 135) -> (295, 165)
  line L72 (295, 165) -> (300, 165)
  line L73 (300, 165) -> (300, 220)
  line L74 (300, 220) -> (295, 220)
  line L75 (295, 220) -> (295, 250)
sketch "left_right" plane through (0, 0, 0) normal (-1, 0, 0) x (0, -1, 0)
  line L0 (-120, 90) -> (-120, 95)
  line L1 (-120, 95) -> (-90, 95)
  line L2 (-90, 95) -> (-90, 90)
  line L3 (-90, 90) -> (-120, 90)
  line L4 (-230, 90) -> (-230, 95)
  line L5 (-230, 95) -> (-200, 95)
  line L6 (-200, 95) -> (-200, 90)
  line L7 (-200, 90) -> (-230, 90)
  line L8 (-120, 180) -> (-120, 185)
  line L9 (-120, 185) -> (-90, 185)
  line L10 (-90, 185) -> (-90, 180)
  line L11 (-90, 180) -> (-120, 180)
  line L12 (-230, 180) -> (-230, 185)
  line L13 (-230, 185) -> (-200, 185)
  line L14 (-200, 185) -> (-200, 180)
  line L15 (-200, 180) -> (-230, 180)
  line L16 (-275, 295) -> (-275, 250)
  line L17 (-275, 250) -> (-280, 250)
  line L18 (-280, 250) -> (-280, 220)
  line L19 (-280, 220) -> (-275, 220)
  line L20 (-275, 220) -> (-275, 165)
  line L21 (-275, 165) -> (-280, 165)
  line L22 (-280, 165) -> (-280, 135)
  line L23 (-280, 135) -> (-275, 135)
  line L24 (-275, 135) -> (-275, 80)
  line L25 (-275, 80) -> (-280, 80)
  line L26 (-280, 80) -> (-280, 50)
  line L27 (-280, 50) -> (-275, 50)
  line L28 (-275, 50) -> (-275, 5)
  line L29 (-275, 5) -> (-250, 5)
  line L30 (-250, 5) -> (-250, 0)
  line L31 (-250, 0) -> (-220, 0)
  line L32 (-220, 0) -> (-220, 5)
  line L33 (-220, 5) -> (-193.3333, 5)
  line L34 (-193.3333, 5) -> (-193.3333, 0)
  line L35 (-193.3333, 0) -> (-163.3333, 0)
  line L36 (-163.3333, 0) -> (-163.3333, 5)
  line L37 (-163.3333, 5) -> (-136.6667, 5)
  line L38 (-136.6667, 5) -> (-136.6667, 0)
  line L39 (-136.6667, 0) -> (-106.6667, 0)
  line L40 (-106.6667, 0) -> (-106.6667, 5)
  line L41 (-106.6667, 5) -> (-80, 5)
  line L42 (-80, 5) -> (-80, 0)
  line L43 (-80, 0) -> (-50, 0)
  line L44 (-50, 0) -> (-50, 5)
  line L45 (-50, 5) -> (-5, 5)
  line L46 (-5, 5) -> (-5, 50)
  line L47 (-5, 50) -> (0, 50)
  line L48 (0, 50) -> (0, 80)
  line L49 (0, 80) -> (-5, 80)
  line L50 (-5, 80) -> (-5, 135)
  line L51 (-5, 135) -> (0, 135)
  line L52 (0, 135) -> (0, 165)
  line L53 (0, 165) -> (-5, 165)
  line L54 (-5, 165) -> (-5, 220)
  line L55 (-5, 220) -> (0, 220)
  line L56 (0, 220) -> (0, 250)
  line L57 (0, 250) -> (-5, 250)
  line L58 (-5, 250) -> (-5, 295)
  line L59 (-5, 295) -> (-50, 295)
  line L60 (-50, 295) -> (-50, 300)
  line L61 (-50, 300) -> (-80, 300)
  line L62 (-80, 300) -> (-80, 295)
  line L63 (-80, 295) -> (-106.6667, 295)
  line L64 (-106.6667, 295) -> (-106.6667, 300)
  line L65 (-106.6667, 300) -> (-136.6667, 300)
  line L66 (-136.6667, 300) -> (-136.6667, 295)
  line L67 (-136.6667, 295) -> (-163.3333, 295)
  line L68 (-163.3333, 295) -> (-163.3333, 300)
  line L69 (-163.3333, 300) -> (-193.3333, 300)
  line L70 (-193.3333, 300) -> (-193.3333, 295)
  line L71 (-193.3333, 295) -> (-220, 295)
  line L72 (-220, 295) -> (-220, 300)
  line L73 (-220, 300) -> (-250, 300)
  line L74 (-250, 300) -> (-250, 295)
  line L75 (-250, 295) -> (-275, 295)
sketch "top_bottom" plane through (0, 0, 300) normal (0, 0, 1) x (-1, 0, 0)
  line L0 (-50, -275) -> (0, -275)
  line L1 (0, -275) -> (0, -250)
  line L2 (0, -250) -> (-5, -250)
  line L3 (-5, -250) -> (-5, -220)
  line L4 (-5, -220) -> (0, -220)
  line L5 (0, -220) -> (0, -193.3333)
  line L6 (0, -193.3333) -> (-5, -193.3333)
  line L7 (-5, -193.3333) -> (-5, -163.3333)
  line L8 (-5, -163.3333) -> (0, -163.3333)
  line L9 (0, -163.3333) -> (0, -136.6667)
  line L10 (0, -136.6667) -> (-5, -136.6667)
  line L11 (-5, -136.6667) -> (-5, -106.6667)
  line L12 (-5, -106.6667) -> (0, -106.6667)
  line L13 (0, -106.6667) -> (0, -80)
  line L14 (0, -80) -> (-5, -80)
  line L15 (-5, -80) -> (-5, -50)
  line L16 (-5, -50) -> (0, -50)
  line L17 (0, -50) -> (0, -5)
  line L18 (0, -5) -> (-50, -5)
  line L19 (-50, -5) -> (-50, 0)
  line L20 (-50, 0) -> (-80, 0)
  line L21 (-80, 0) -> (-80, -5)
  line L22 (-80, -5) -> (-106.6667, -5)
  line L23 (-106.6667, -5) -> (-106.6667, 0)
  line L24 (-106.6667, 0) -> (-136.6667, 0)
  line L25 (-136.6667, 0) -> (-136.6667, -5)
  line L26 (-136.6667, -5) -> (-163.3333, -5)
  line L27 (-163.3333, -5) -> (-163.3333, 0)
  line L28 (-163.3333, 0) -> (-193.3333, 0)
  line L29 (-193.3333, 0) -> (-193.3333, -5)
  line L30 (-193.3333, -5) -> (-220, -5)
  line L31 (-220, -5) -> (-220, 0)
  line L32 (-220, 0) -> (-250, 0)
  line L33 (-250, 0) -> (-250, -5)
  line L34 (-250, -5) -> (-300, -5)
  line L35 (-300, -5) -> (-300, -50)
  line L36 (-300, -50) -> (-295, -50)
  line L37 (-295, -50) -> (-295, -80)
  line L38 (-295, -80) -> (-300, -80)
  line L39 (-300, -80) -> (-300, -106.6667)
  line L40 (-300, -106.6667) -> (-295, -106.6667)
  line L41 (-295, -106.6667) -> (-295, -136.6667)
  line L42 (-295, -136.6667) -> (-300, -136.6667)
  line L43 (-300, -136.6667) -> (-300, -163.3333)
  line L44 (-300, -163.3333) -> (-295, -163.3333)
  line L45 (-295, -163.3333) -> (-295, -193.3333)
  line L46 (-295, -193.3333) -> (-300, -193.3333)
  line L47 (-300, -193.3333) -> (-300, -220)
  line L48 (-300, -220) -> (-295, -220)
  line L49 (-295, -220) -> (-295, -250)
  line L50 (-295, -250) -> (-300, -250)
  line L51 (-300, -250) -> (-300, -275)
  line L52 (-300, -275) -> (-250, -275)
  line L53 (-250, -275) -> (-250, -280)
  line L54 (-250, -280) -> (-220, -280)
  line L55 (-220, -280) -> (-220, -275)
  line L56 (-220, -275) -> (-193.3333, -275)
  line L57 (-193.3333, -275) -> (-193.3333, -280)
  line L58 (-193.3333, -280) -> (-163.3333, -280)
  line L59 (-163.3333, -280) -> (-163.3333, -275)
  line L60 (-163.3333, -275) -> (-136.6667, -275)
  line L61 (-136.6667, -275) -> (-136.6667, -280)
  line L62 (-136.6667, -280) -> (-106.6667, -280)
  line L63 (-106.6667, -280) -> (-106.6667, -275)
  line L64 (-106.6667, -275) -> (-80, -275)
  line L65 (-80, -275) -> (-80, -280)
  line L66 (-80, -280) -> (-50, -280)
  line L67 (-50, -280) -> (-50, -275)
sketch "back" plane through (0, 280, 0) normal (0, 1, 0) x (-1, 0, 0)
  line L0 (-300, 250) -> (-295, 250)
  line L1 (-295, 250) -> (-295, 220)
  line L2 (-295, 220) -> (-300, 220)
  line L3 (-300, 220) -> (-300, 165)
  line L4 (-300, 165) -> (-295, 165)
  line L5 (-295, 165) -> (-295, 135)
  line L6 (-295, 135) -> (-300, 135)
  line L7 (-300, 135) -> (-300, 80)
  line L8 (-300, 80) -> (-295, 80)
  line L9 (-295, 80) -> (-295, 50)
  line L10 (-295, 50) -> (-300, 50)
  line L11 (-300, 50) -> (-300, 0)
  line L12 (-300, 0) -> (-250, 0)
  line L13 (-250, 0) -> (-250, 5)
  line L14 (-250, 5) -> (-220, 5)
  line L15 (-220, 5) -> (-220, 0)
  line L16 (-220, 0) -> (-193.3333, 0)
  line L17 (-193.3333, 0) -> (-193.3333, 5)
  line L18 (-193.3333, 5) -> (-163.3333, 5)
  line L19 (-163.3333, 5) -> (-163.3333, 0)
  line L20 (-163.3333, 0) -> (-136.6667, 0)
  line L21 (-136.6667, 0) -> (-136.6667, 5)
  line L22 (-136.6667, 5) -> (-106.6667, 5)
  line L23 (-106.6667, 5) -> (-106.6667, 0)
  line L24 (-106.6667, 0) -> (-80, 0)
  line L25 (-80, 0) -> (-80, 5)
  line L26 (-80, 5) -> (-50, 5)
  line L27 (-50, 5) -> (-50, 0)
  line L28 (-50, 0) -> (0, 0)
  line L29 (0, 0) -> (0, 50)
  line L30 (0, 50) -> (-5, 50)
  line L31 (-5, 50) -> (-5, 80)
  line L32 (-5, 80) -> (0, 80)
  line L33 (0, 80) -> (0, 135)
  line L34 (0, 135) -> (-5, 135)
  line L35 (-5, 135) -> (-5, 165)
  line L36 (-5, 165) -> (0, 165)
  line L37 (0, 165) -> (0, 220)
  line L38 (0, 220) -> (-5, 220)
  line L39 (-5, 220) -> (-5, 250)
  line L40 (-5, 250) -> (0, 250)
  line L41 (0, 250) -> (0, 300)
  line L42 (0, 300) -> (-50, 300)
  line L43 (-50, 300) -> (-50, 295)
  line L44 (-50, 295) -> (-80, 295)
  line L45 (-80, 295) -> (-80, 300)
  line L46 (-80, 300) -> (-106.6667, 300)
  line L47 (-106.6667, 300) -> (-106.6667, 295)
  line L48 (-106.6667, 295) -> (-136.6667, 295)
  line L49 (-136.6667, 295) -> (-136.6667, 300)
  line L50 (-136.6667, 300) -> (-163.3333, 300)
  line L51 (-163.3333, 300) -> (-163.3333, 295)
  line L52 (-163.3333, 295) -> (-193.3333, 295)
  line L53 (-193.3333, 295) -> (-193.3333, 300)
  line L54 (-193.3333, 300) -> (-220, 300)
  line L55 (-220, 300) -> (-220, 295)
  line L56 (-220, 295) -> (-250, 295)
  line L57 (-250, 295) -> (-250, 300)
  line L58 (-250, 300) -> (-300, 300)
  line L59 (-300, 300) -> (-300, 250)
sketch "divider" plane through (113.0378, 0, 0) normal (1, 0, 0) x (0, 1, 0)
  line L0 (60, 95) -> (240, 95)
  line L1 (240, 95) -> (240, 140)
  line L2 (240, 140) -> (245, 140)
  line L3 (245, 140) -> (245, 170)
  line L4 (245, 170) -> (240, 170)
  line L5 (240, 170) -> (240, 180)
  line L6 (240, 180) -> (189.9998, 180)
  line L7 (189.9998, 180) -> (189.9998, 185)
  line L8 (189.9998, 185) -> (240, 185)
  line L9 (240, 185) -> (240, 196)
  line L10 (240, 196) -> (245, 196)
  line L11 (245, 196) -> (245, 226)
  line L12 (245, 226) -> (240, 226)
  line L13 (240, 226) -> (240, 265)
  line L14 (240, 265) -> (60, 265)
  line L15 (60, 265) -> (60, 185)
  line L16 (60, 185) -> (129.9998, 185)
  line L17 (129.9998, 185) -> (129.9998, 180)
  line L18 (129.9998, 180) -> (60, 180)
  line L19 (60, 180) -> (60, 95)
sketch "supporting_1" plane through (0, 0, 95) normal (0, 0, 1) x (-1, 0, 0)
  line L0 (-112.0378, -230) -> (-112.0378, -200)
  line L1 (-112.0378, -200) -> (-107.0378, -200)
  line L2 (-107.0378, -200) -> (-107.0378, -230)
  line L3 (-107.0378, -230) -> (-112.0378, -230)
  line L4 (-295, -260) -> (-5, -260)
  line L5 (-5, -260) -> (-5, -230)
  line L6 (-5, -230) -> (1, -230)
  line L7 (1, -230) -> (1, -200)
  line L8 (1, -200) -> (-5, -200)
  line L9 (-5, -200) -> (-5, -160)
  line L10 (-5, -160) -> (-295, -160)
  line L11 (-295, -160) -> (-295, -200)
  line L12 (-295, -200) -> (-301, -200)
  line L13 (-301, -200) -> (-301, -230)
  line L14 (-301, -230) -> (-295, -230)
  line L15 (-295, -230) -> (-295, -260)
sketch "supporting_2" plane through (0, 0, 185) normal (0, 0, 1) x (-1, 0, 0)
  line L0 (-5, -200) -> (-5, -160)
  line L1 (-5, -160) -> (-108.0378, -160)
  line L2 (-108.0378, -160) -> (-108.0378, -189.9998)
  line L3 (-113.0378, -189.9998) -> (-113.0378, -160)
  line L4 (-295, -160) -> (-295, -200)
  line L5 (-295, -200) -> (-300, -200)
  line L6 (-300, -200) -> (-300, -230)
  line L7 (-300, -230) -> (-295, -230)
  line L8 (-295, -230) -> (-295, -240)
  line L9 (-108.0378, -240) -> (-5, -240)
  line L10 (-5, -240) -> (-5, -230)
  line L11 (-5, -230) -> (0, -230)
  line L12 (0, -230) -> (0, -200)
  line L13 (0, -200) -> (-5, -200)
  line L14 (-295, -240) -> (-113.0378, -240)
  line L15 (-113.0378, -160) -> (-295, -160)
  line L16 (-108.0378, -189.9998) -> (-113.0378, -189.9998)
  line L17 (-113.0378, -240) -> (-108.0378, -240)
sketch "supporting_3" plane through (0, 0, 185) normal (0, 0, 1) x (-1, 0, 0)
  line L0 (-295, -60) -> (-295, -90)
  line L1 (-295, -90) -> (-300, -90)
  line L2 (-300, -90) -> (-300, -120)
  line L3 (-300, -120) -> (-295, -120)
  line L4 (-295, -120) -> (-295, -160)
  line L5 (-108.0378, -160) -> (-5, -160)
  line L6 (-113.0378, -160) -> (-113.0378, -129.9998)
  line L7 (-108.0378, -129.9998) -> (-108.0378, -160)
  line L8 (-5, -160) -> (-5, -120)
  line L9 (-5, -120) -> (0, -120)
  line L10 (0, -120) -> (0, -90)
  line L11 (0, -90) -> (-5, -90)
  line L12 (-5, -90) -> (-5, -60)
  line L13 (-113.0378, -60) -> (-295, -60)
  line L14 (-295, -160) -> (-113.0378, -160)
  line L15 (-5, -60) -> (-108.0378, -60)
  line L16 (-113.0378, -129.9998) -> (-108.0378, -129.9998)
  line L17 (-108.0378, -60) -> (-113.0378, -60)
sketch "motor-holder" plane through (0, 240, 0) normal (0, -1, 0) x (1, 0, 0)
  line L0 (170, 240) -> (50, 240)
  line L1 (50, 240) -> (50, 110)
  line L2 (50, 110) -> (170, 110)
  line L3 (170, 110) -> (170, 240)
  line L4 (107.0378, 225) -> (112.0378, 225)
  line L5 (112.0378, 225) -> (112.0378, 195)
  line L6 (112.0378, 195) -> (107.0378, 195)
  line L7 (107.0378, 195) -> (107.0378, 225)
  line L8 (112.0378, 125) -> (107.0378, 125)
  line L9 (107.0378, 125) -> (107.0378, 155)
  line L10 (107.0378, 155) -> (112.0378, 155)
  line L11 (112.0378, 155) -> (112.0378, 125)
  line L12 (143.5, 197.5) -> (143.5, 222.5)
  line L13 (143.5, 222.5) -> (156.5, 222.5)
  line L14 (156.5, 222.5) -> (156.5, 197.5)
  line L15 (156.5, 197.5) -> (143.5, 197.5)
  line L16 (63.5, 117.5) -> (63.5, 142.5)
  line L17 (63.5, 142.5) -> (76.5, 142.5)
  line L18 (76.5, 142.5) -> (76.5, 117.5)
  line L19 (76.5, 117.5) -> (63.5, 117.5)
  line L20 (63.5, 222.5) -> (76.5, 222.5)
  line L21 (76.5, 222.5) -> (76.5, 197.5)
  line L22 (76.5, 197.5) -> (63.5, 197.5)
  line L23 (63.5, 197.5) -> (63.5, 222.5)
  line L24 (143.5, 117.5) -> (143.5, 142.5)
  line L25 (143.5, 142.5) -> (156.5, 142.5)
  line L26 (156.5, 142.5) -> (156.5, 117.5)
  line L27 (156.5, 117.5) -> (143.5, 117.5)
combine "Combine18" operation add target body 11 tool bodies 7
hidden bodies 8 9 10
equation "Thickness = 5 mm"
equation "Base = 30 cm"
equation "Height = 30 cm"
equation "Width = 28 cm"
equation "d9 = Base"
equation "d10 = Height"
equation "d11 = Thickness"
equation "d13 = Base"
equation "d14 = Width"
equation "support_width = 20 cm"
equation "divider_height = 6 cm"
equation "divider_width = 20 cm"
equation "opening_base = 16 cm"
equation "opening_height = 6 cm"
equation "box_base = 10 cm"
equation "box_height = 6.5 cm"
equation "box_width = 6 cm"
equation "finger_base = 30 mm"
equation "finger_height = Thickness"
equation "d28 = finger_base"
equation "d29 = finger_height"
equation "d32 = finger_base"
equation "d33 = finger_height"
equation "d34 = Thickness"
equation "d42 = Base"
equation "d43 = Width"
equation "d44 = Thickness"
equation "d48 = finger_height"
equation "d49 = finger_base"
equation "d50 = Thickness"
equation "d63 = finger_height"
equation "d64 = finger_base"
equation "d65 = Thickness"
equation "d75 = Width"
equation "d76 = Height"
equation "d77 = Thickness"
equation "d81 = opening_base"
equation "d82 = opening_height"
equation "d83 = -Thickness"
equation "d85 = opening_base"
equation "d87 = -Thickness"
equation "d115 = Base - 10 mm"
equation "d116 = support_width"
equation "d117 = finger_height + 1 mm"
equation "d118 = finger_base"